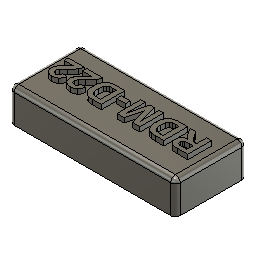
wali_magnet_template (Autodesk Fusion 360 design; units mm, degrees)
Autodesk Fusion 360 part; units mm, degrees
sketch "Sketch1" plane through (0, 0, 0) normal (0, 1, 0) x (1, 0, 0)
  line L0 (17.5, -7.5) -> (-17.5, -7.5)
  line L1 (-17.5, -7.5) -> (-17.5, 7.5)
  line L2 (-17.5, 7.5) -> (17.5, 7.5)
  line L3 (17.5, 7.5) -> (17.5, -7.5)
  line L4 (17.5, -7.5) -> (-17.5, 7.5) construction
  line L5 (-17.5, -7.5) -> (17.5, 7.5) construction
  dimension "d1" = 35
  dimension "d2" = 15
  constraint horizontal L0
  constraint perpendicular L0 L1
  constraint parallel L0 L2
  constraint parallel L1 L3
  constraint coincident L4 origin
  constraint coincident L5 origin
  measures "d1" distance of L1.end L2.end
  measures "d2" distance of L0.end L1.end
extrude "Extrude1" add sketch "Sketch1" along normal blind 7
hole "Hole1" at (0, 0, 0) direction (0, 1, 0) diameter 8 depth 4 tip angle 180
fillet "Fillet1" radius 1 8 edges at (17.5, 7, 0) (0, 7, 7.5) (-17.5, 7, 0) (0, 7, -7.5) (-17.5, 3.5, -7.5) (-17.5, 3.5, 7.5) (17.5, 3.5, -7.5) (17.5, 3.5, 7.5)
sketch "wali-text" plane through (0, 7, 0) normal (0, 1, 0) x (-1, 0, 0)
  line L0 (-16.5, -6.5) -> (16.5, -6.5)
  line L1 (16.5, -6.5) -> (16.5, 6.5)
  line L2 (16.5, 6.5) -> (-16.5, 6.5)
  line L3 (-16.5, 6.5) -> (-16.5, -6.5)
  line L4 (-13, -6) -> (13, -6) construction
  line L5 (13, -6) -> (13, 6) construction
  line L6 (13, 6) -> (-13, 6) construction
  line L7 (-13, 6) -> (-13, -6) construction
  dimension "d17" = 5
  text T0 "RDM-D22" font "Arial" height 5 bold align centre middle in box 26 x 12 at (-13, -6) x (1, 0) y (0, 1) spacing 1
extrude "Extrude2" add sketch "wali-text" along normal blind 1 text T0
equation "d1 = rect_width"
equation "d2 = rect_height"
equation "rect_width = 35 mm"
equation "rect_height = 15 mm"
equation "rect_thickness = 7 mm"
equation "magnet_diameter = 6 mm"
equation "magnet_thickness = 3 mm"
equation "magnet_clearance = 1 mm" comment "Includes extra space for glue"
equation "d9 = rect_thickness"
equation "d11 = magnet_thickness + magnet_clearance"
equation "d12 = magnet_diameter + 2 * magnet_clearance"
equation "fillet_radius = 1 mm"
equation "d16 = fillet_radius"
equation "d17 = text_height"
equation "text_height = 5 mm"
equation "text_emboss_depth = 1 mm"
equation "d20 = text_emboss_depth"
